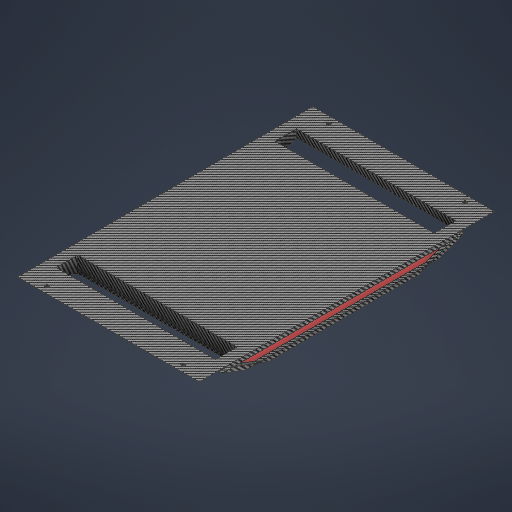
# Autodesk Inventor part: Top Cover
Saved by Autodesk Inventor 2026.1 (Build 301233000, 233)
## iProperties
Created: 2026-07-14
Part Number: Top Cover
Material: Generic
Document SubType Name: Modeling
Designer: ankit
Density: 1 g/cm^3
Appearance: Default
Author: ankit
Autodesk Inventor part; units mm, degrees
ref_plane "YZ Plane" through (0, 0, 0) normal (1, 0, 0) x (0, 1, 0)
ref_plane "XZ Plane" through (0, 0, 0) normal (0, 1, 0) x (-1, 0, 0)
ref_plane "XY Plane" through (0, 0, 0) normal (0, 0, 1) x (1, 0, 0)
sketch "Sketch1" plane through (0, 0, 0) normal (0, 1, 0) x (-1, 0, 0)
  line L0 (80, 130) -> (-80, 130)
  line L1 (-80, 130) -> (-80, -130)
  line L2 (-80, -130) -> (80, -130)
  line L3 (80, -130) -> (80, 130)
  line L4 (80, 130) -> (-80, -130) construction
  line L5 (-80, 130) -> (80, -130) construction
  line L6 (80, 130) -> (67.5, 130)
  line L7 (67.5, 130) -> (52.5, 130)
  line L8 (52.5, 130) -> (52.5, 118)
  line L9 (52.5, 118) -> (67.5, 118)
  line L10 (67.5, 118) -> (67.5, 130)
  line L11 (0, 130) -> (0, -130)
  line L12 (80, 0) -> (-80, 0)
  circle A0 centre (60, 124) radius 1.5
  line L13 (67.5, 130) -> (52.5, 130)
  line L14 (80, -130) -> (-80, -130)
  line L15 (80, -130) -> (-80, 130) construction
  line L16 (80, -130) -> (67.5, -130)
  line L17 (52.5, -130) -> (52.5, -118)
  line L18 (52.5, -118) -> (67.5, -118)
  line L19 (67.5, -118) -> (67.5, -130)
  circle A1 centre (60, -124) radius 1.5
  line L20 (-67.5, 130) -> (-52.5, 130)
  line L21 (-52.5, 118) -> (-67.5, 118)
  line L22 (-67.5, 118) -> (-67.5, 130)
  circle A2 centre (-60, 124) radius 1.5
  line L23 (-67.5, 130) -> (-52.5, 130)
  line L24 (-52.5, -130) -> (-52.5, -118)
  line L25 (-67.5, -118) -> (-67.5, -130)
  line L26 (-52.5, -118) -> (-67.5, -118)
  circle A3 centre (-60, -124) radius 1.5
  line L27 (-80, 130) -> (-67.5, 130)
  line L28 (-52.5, 118) -> (-52.5, 130)
  point P0 (0, 0)
  dimension "d0" = 160
  dimension "d1" = 260
  dimension "d14" = 12
  dimension "d15" = 15
  dimension "d16" = 12.5
  constraints: 58 end point, 17 symmetric about line, 6 midpoint, 4 centre point, 4 parallel, 4 point on line, 3 perpendicular, 2 horizontal, 1 collinear, 3 other
  measures "d0" distance of L2.end L1.end
  measures "d1" distance of L1.end L0.end
  measures "d14" distance of L20.end L21.start
  measures "d15" distance of L21.start L21.end
  measures "d16" distance of L15.end L27.end
extrude "Extrusion1" add sketch "Sketch1" along normal blind 3
chamfer "Chamfer1" distance 3 angle 45 4 edges at (0, 0, -130) (0, 0, 130) (-80, 0, 0) (80, 0, 0)
sketch "Sketch2" plane through (0, 0, 0) normal (0, -1, 0) x (1, 0, 0)
  line L0 (-77, -127) -> (-77, 127) projected
  line L1 (77, 116.0107) -> (-77, 116.0107)
  line L2 (-77, 116.0107) -> (-77, -116.0107)
  line L3 (-77, -116.0107) -> (77, -116.0107)
  line L4 (77, -116.0107) -> (77, 116.0107)
  line L5 (77, 116.0107) -> (-77, -116.0107) construction
  line L6 (-77, 116.0107) -> (77, -116.0107) construction
  point P0 (0, 0)
  constraints: 12 end point, 2 midpoint, 2 parallel, 1 horizontal, 1 perpendicular, 1 point on line
extrude "Extrusion2" add sketch "Sketch2" along normal blind 50
sketch "Sketch4" plane through (-77, -50, -116.0107) normal (-1, 0, 0) x (0, 0, 1)
  line L0 (232.0214, 50) -> (232.0214, 0) projected
  line L1 (246.0107, 53) -> (-13.9893, 53) projected
  line L2 (232.0214, 50) -> (192.0214, 50)
  line L3 (0, 50) -> (232.0214, 50) projected
  line L4 (192.0214, 50) -> (192.0214, 35)
  line L5 (192.0214, 35) -> (232.0214, 50)
  line L6 (0, 50) -> (40, 50)
  line L7 (40, 50) -> (40, 35)
  line L8 (40, 35) -> (0, 50)
  line L9 (40, 35) -> (192.0214, 35)
  line L10 (232.0214, 0) -> (0, 0) projected
  line L11 (0, 50) -> (0, 0)
  line L12 (0, 0) -> (232.0214, 0)
  line L13 (232.0214, 0) -> (232.0214, 50)
  point P0 (116.0107, 50)
  dimension "d21" = 40
  dimension "d22" = 15
  dimension "d23" = 40
  constraints: 20 end point, 4 perpendicular, 2 point on line, 1 collinear, 1 vertical
  measures "d21" distance of L0.start L2.end
  measures "d22" distance of L2.end L4.end
  measures "d23" distance of L3.start L6.end
extrude "Extrusion3" cut sketch "Sketch4" against normal through all contours L0 L10 L11 L8 L9 L5
sketch "Sketch5" plane through (-77, -15, -76.0107) normal (0, -1, 0) x (1, 0, 0)
  point P0 (77, 76.0107)
sketch "Sketch6" plane through (77, 0, 116.0107) normal (1, 0, 0) x (0, 0, -1)
  line L0 (192.0214, -15) -> (232.0214, 0) projected
  line L1 (232.0214, 0) -> (222.0214, 0)
  line L2 (0, 0) -> (232.0214, 0) projected
  line L3 (232.0214, 0) -> (192.0214, -15)
  line L4 (192.0214, -15) -> (182.0214, -15)
  line L5 (192.0214, -15) -> (40, -15) projected
  line L6 (182.0214, -15) -> (222.0214, 0)
  line L7 (192.0214, -15) -> (201.3847, -11.4888)
  line L8 (40, -15) -> (30.6367, -11.4888)
  line L9 (40, -15) -> (0, 0) projected
  line L10 (30.6367, -11.4888) -> (201.3847, -11.4888)
  line L11 (232.0214, 0) -> (222.6581, -3.5112)
  line L12 (0, 0) -> (9.3633, -3.5112)
  line L13 (0, 0) -> (10, 0)
  line L14 (40, -15) -> (50, -15)
  line L15 (50, -15) -> (10, 0)
  line L16 (9.3633, -3.5112) -> (222.6581, -3.5112)
  point P0 (116.0107, 0)
  point P1 (212.6581, -3.5112)
  point P2 (19.3633, -3.5112)
  point P3 (40.6367, -11.4888)
  point P4 (191.3847, -11.4888)
  dimension "d26" = 10
  dimension "d27" = 10
  dimension "d28" = 10
  dimension "d29" = 10
  dimension "d30" = 10
  dimension "d31" = 10
  dimension "d32" = 10
  dimension "d33" = 10
  constraints: 26 end point, 9 point on line, 1 collinear, 1 horizontal
  measures "d26" distance of L0.end L1.end
  measures "d27" distance of L0.start L4.end
  measures "d28" distance of L0.start L7.end
  measures "d29" distance of L5.end L8.end
  measures "d30" distance of L0.end L11.end
  measures "d31" distance of L2.start L12.end
  measures "d32" distance of L2.start L13.end
  measures "d33" distance of L5.end L14.end
extrude "Extrusion4" cut sketch "Sketch6" against normal blind 3 contours L4 L6 L10 L0 | L16 L6 L1 L0 | L10 L15 L16 L6 | L5 L8 L10 L15 | L16 L9 L2 L15
mirror "Mirror1" about plane through (0, 0, 0) normal (1, 0, 0) of "Extrusion4"
sketch "Sketch7" plane through (77, -15, -66.0107) normal (0, -1, 0) x (1, 0, 0)
  line L0 (-154, 0) -> (-151, 0) projected
  line L1 (-151, 0) -> (-151, 132.0214)
  line L2 (-151, 132.0214) -> (-3, 132.0214)
  line L3 (-3, 132.0214) -> (-3, 0)
  line L4 (-3, 0) -> (-151, 0)
  line L5 (-135, 11.0214) -> (-19, 11.0214)
  line L6 (-19, 11.0214) -> (-19, 121)
  line L7 (-19, 121) -> (-135, 121)
  line L8 (-135, 121) -> (-135, 11.0214)
  line L9 (-135, 11.0214) -> (-19, 121) construction
  line L10 (-19, 11.0214) -> (-135, 121) construction
  point P0 (-77, 66.0107)
  constraints: 20 end point, 4 perpendicular, 2 midpoint, 2 parallel, 1 horizontal, 1 vertical
extrude "Extrusion5" cut sketch "Sketch7" against normal blind 5 contours L8 L7 L6 L5
chamfer "Chamfer2" distance 5 angle 45 4 edges at (0, -15, -54.9893) (0, -15, 54.9893) (58, -15, 0) (-58, -15, 0)
sketch "Sketch8" plane through (-74, 0, -116.0107) normal (0, -0.9363292, -0.3511234) x (1, 0, 0)
  line L0 (0, 32.72) -> (-3, 32.72) projected
  line L1 (148, 9.3633) -> (148, 0) projected
  line L2 (0, 32.72) -> (148, 32.72)
  line L3 (148, 32.72) -> (148, 9.3633)
  line L4 (148, 9.3633) -> (0, 9.3633)
  line L5 (0, 9.3633) -> (0, 32.72)
  line L6 (4, 31.0417) -> (144, 31.0417)
  line L7 (144, 31.0417) -> (144, 11.0417)
  line L8 (144, 11.0417) -> (4, 11.0417)
  line L9 (4, 11.0417) -> (4, 31.0417)
  line L10 (4, 31.0417) -> (144, 11.0417) construction
  line L11 (144, 31.0417) -> (4, 11.0417) construction
  point P0 (74, 108.6242)
  point P1 (74, 21.0417)
  dimension "d41" = 140
  dimension "d42" = 20
  constraints: 20 end point, 4 parallel, 2 horizontal, 2 midpoint, 2 perpendicular
  measures "d41" distance of L7.end L8.end
  measures "d42" distance of L6.end L7.end
extrude "Extrusion6" cut sketch "Sketch8" against normal blind 3 contours L6 L7 L8 L9
mirror "Mirror2" about plane through (0, 0, 0) normal (0, 0, 1) of "Extrusion6"
thread "Thread1" size "M3x0.5" class "6H" standard "ANSI Metric M Profile" full length
thread "Thread2" size "M3x0.5" class "6H" standard "ANSI Metric M Profile" full length
thread "Thread3" size "M3x0.5" class "6H" standard "ANSI Metric M Profile" full length
thread "Thread4" size "M3x0.5" class "6H" standard "ANSI Metric M Profile" full length
sketch "Sketch9" plane through (77, -10, -66.0107) normal (0, -1, 0) x (1, 0, 0)
  line L0 (-147, 171.6828) -> (-7, 171.6828) projected
  line L1 (-7, 152.9562) -> (-7, 151.9028) projected
  line L2 (-7, 171.6828) -> (-7, 152.9562)
  line L3 (-7, 152.9562) -> (-147, 152.9562)
  line L4 (-147, 151.9028) -> (-7, 151.9028) projected
  line L5 (-147, 152.9562) -> (-147, 171.6828)
  line L6 (-147, 171.6828) -> (-7, 171.6828)
  line L7 (-157, 196.0107) -> (3, 196.0107) projected
  line L8 (0, -60.9893) -> (3, -63.9893) projected
  line L9 (3, 196.0107) -> (3, -63.9893)
  line L10 (3, -63.9893) -> (3, 66.0107)
  line L11 (3, 66.0107) -> (-163, 66.0107)
  line L12 (-147, -39.6614) -> (-7, -39.6614)
  line L13 (-7, -39.6614) -> (-7, -20.9348)
  line L14 (-7, -20.9348) -> (-147, -20.9348)
  line L15 (-147, -20.9348) -> (-147, -39.6614)
  point P0 (-77, 66.0107)
  constraints: 22 end point, 5 symmetric about line, 2 perpendicular, 1 collinear, 1 horizontal, 1 midpoint, 1 parallel, 1 vertical
extrude "Extrusion7" cut sketch "Sketch9" against normal through all
fillet "Fillet3" radius 2 2 edges at (0, -7.6933, 86.9455) (0, -8.0886, 85.8914)
fillet "Fillet4" radius 2 2 edges at (0, -7.6933, -86.9455) (0, -8.0886, -85.8914)
body "Solid1"
